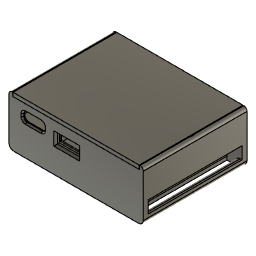
case 8.0 v12 (Autodesk Fusion 360 design; units mm, degrees)
Autodesk Fusion 360 part; units mm, degrees
note: some values were not read from the file. Chosen so that the rebuilt part matches the saved one: which bodies a step acts on; which face or edge a step refers to. Set by a fixed rule: which sketch regions a step uses.
sketch "battery base" plane through (0, 0, 0) normal (0, 0, 1) x (1, 0, 0) in component "case"
  line L0 (0, 0) -> (41, 0)
  line L1 (41, 0) -> (41, 41)
  line L2 (41, 41) -> (0, 41)
  line L3 (0, 41) -> (0, 0)
  dimension "d1" = 41
  dimension "d2" = 41
  constraint horizontal L0
  constraint vertical L1
  constraint horizontal L2
  constraint vertical L3
  constraint coincident L0.start L3.end
  measures "d1" distance of L0.start L2.end
  measures "d2" distance of L0.start L0.end
extrude "Extrude1" add sketch "battery base" along normal blind 8.6 makes body 1 in component "case"
sketch "tray base" plane through (0, 0, 8.6) normal (0, 0, 1) x (-1, 0, 0) in component "case"
  line L0 (0, -41) -> (0, 0)
  line L1 (0, 0) -> (-41, 0)
  line L2 (-41, 0) -> (-41, -41)
  line L3 (-41, -41) -> (0, -41)
  line L4 (-41, -41) -> (-47.5, -41)
  line L5 (-47.5, -41) -> (-47.5, 0)
  line L6 (-47.5, 0) -> (-41, 0)
  line L7 (-20.5, 0) -> (-20.5, -41) construction
  line L8 (6.5, -41) -> (6.5, 0)
  line L9 (6.5, 0) -> (0, 0)
  line L10 (0, -41) -> (6.5, -41)
  point P0 (18.675, 37.8)
  dimension "d5" = 6.5
  constraint coincident L2.end L3.start
  constraint perpendicular L2 L4
  constraint perpendicular L1 L5
  constraint coincident L1.end L2.start
  constraint perpendicular L2 L6
  constraint midpoint L1 L7.start
  constraint midpoint L3 L7.end
  constraint symmetric L2.end L7 L0.start
  constraint symmetric L4.end L7 L8.start
  constraint symmetric L5.end L7 L8.end
  constraint symmetric L1.end L7 L0.end
  measures "d5" distance of L5.end L1.end
extrude "Extrude2" add sketch "tray base" along normal blind 9.8 bodies 1 in component "case"
shell "Shell1" thickness 1.6 outward yes removed faces 1 at (11.5, 13.6667, 18.4) on bodies 1 in component "case"
ref_plane "WorkPlane1" through (20.5, 20.5, 8.4) normal (0, -1, 0) x (1, 0, 0) in component "case"
ref_plane "WorkPlane2" through (20.5, 20.5, 2.7) normal (-1, 0, 0) x (0, -1, 0) in component "case"
sketch "buckle" plane through (0, -1.6, 0) normal (0, -1, 0) x (1, 0, 0) in component "case"
  line L0 (42.6, -1.6) -> (49.1, -1.6) construction
  line L1 (49.1, -1.6) -> (49.1, 7) construction
  line L2 (49.1, 1.8) -> (46.3, 1.8) construction
  line L3 (46.3, 1.8) -> (46.3, -1.6) construction
  line L4 (49.1, 1.8) -> (48.3, 1.8)
  line L5 (46.3, -0.2) -> (46.3, -1.6)
  line L6 (46.3, -1.6) -> (47.1, -1.6)
  line L7 (49.1, 0.4) -> (49.1, 1.8)
  arc A0 (47.1, -1.6) -> (49.1, 0.4) centre (47.1, 0.4) ccw
  arc A1 (48.3, 1.8) -> (46.3, -0.2) centre (48.3, -0.2) ccw
  line L8 (-1.6, -1.6) -> (42.6, -1.6)
  line L9 (42.6, -1.6) -> (42.6, 7)
  line L10 (42.6, 7) -> (49.1, 7)
  line L11 (49.1, 7) -> (49.1, 18.4)
  line L12 (49.1, 18.4) -> (-8.1, 18.4)
  line L13 (-8.1, 18.4) -> (-8.1, 7)
  line L14 (-8.1, 7) -> (-1.6, 7)
  line L15 (-1.6, 7) -> (-1.6, -1.6)
  line L16 (49.1, 1.8) -> (49.1, 7)
  line L17 (42.6, -1.6) -> (42.6, 7)
  line L18 (42.6, 7) -> (49.1, 7)
  arc A2 (49.1, 7) -> (42.6, -0.129) centre (50.5661, -0.8645) ccw
  line L19 (42.6, -1.6) -> (46.3, -1.6)
  dimension "d16" = 2
  dimension "d231" = 8
  dimension "d233" = 3.4
  dimension "d234" = 2.8
  constraint coincident L1.end L10.end
  constraint coincident L1 L2.start
  constraint perpendicular L1 L2
  constraint coincident L0 L3.end
  constraint perpendicular L0 L3
  constraint horizontal L4
  constraint vertical L5
  constraint horizontal L6
  constraint vertical L7
  constraint tangent L6 A0
  constraint tangent L7 A0
  constraint tangent L4 A1
  constraint tangent L5 A1
  constraint equal A0 A1
  constraint coincident L0.start L8.end
  constraint coincident L9.end L10.start
  constraint coincident L9 A2.end
  constraint perpendicular L16 L18
  constraint perpendicular L17 L19
  measures "d16" radius of A0
  measures "d231" radius of A2
  measures "d233" distance of L0 L2
  measures "d234" distance of L1 L3
extrude "Extrude1'" add sketch "buckle" against normal up to surface (22.1 mm away) contours L4 L5 L6 L7 A0 A1 | L4 L5 A1 L9 L16 L17 A2 L19 | L9 L10 L17 L18 A2 bodies 1 in component "case"
extrude "Extrude2'" cut sketch "buckle" along normal blind 20 from surface at -22.1 contours L4 L5 A1 L9 L16 L17 A2 L19 bodies 1 in component "case"
mirror "Mirror1" about plane through (20.5, 20.5, 8.4) normal (0, -1, 0) of "Extrude1'", "Extrude2'" in component "case"
split "Split1" by curves path "buckle" along L17 L18 bodies 1 makes body 2 at (13.1333, 27.1667, -1.6) in component "case"
mirror "Mirror2" about plane through (20.5, 20.5, 2.7) normal (-1, 0, 0) of bodies 1 makes body 3 in component "case"
combine "Combine1" operation add target body 2 tool bodies 1 3 in component "case"
sketch "tray" plane through (0, 0, 0) normal (0, 0, 1) x (1, 0, 0) in component "tray"
  line L0 (0, 41) -> (-6.5, 41) construction
  line L1 (41, 41) -> (0, 41) construction
  line L2 (47.5, 41) -> (41, 41) construction
  line L3 (41, 0) -> (47.5, 0) construction
  line L4 (0, 0) -> (41, 0) construction
  line L5 (-6.5, 0) -> (0, 0) construction
  line L6 (-6.5, 41) -> (-6.5, 0) construction
  line L7 (47.5, 41) -> (47.5, 0) construction
  line L8 (41, 0.15) -> (47.35, 0.15)
  line L9 (47.35, 40.85) -> (47.35, 0.15)
  line L10 (47.35, 40.85) -> (41, 40.85)
  line L11 (41, 40.85) -> (0, 40.85)
  line L12 (0, 40.85) -> (-6.35, 40.85)
  line L13 (-6.35, 40.85) -> (-6.35, 0.15)
  line L14 (-6.35, 0.15) -> (0, 0.15)
  line L15 (0, 0.15) -> (41, 0.15)
  line L16 (10.9, 0.15) -> (10.9, 28.4)
  line L17 (10.9, 28.4) -> (-6.35, 28.4)
  line L18 (11.9, 30.6) -> (11.9, 9.7)
  line L19 (11.9, 9.7) -> (27.9, 9.7)
  line L20 (-6.35, 38.6) -> (17.05, 38.6)
  line L21 (-6.35, 38.6) -> (-6.35, 37.8)
  line L22 (-6.35, 37.8) -> (-2.55, 37.8)
  line L23 (-2.55, 37.8) -> (-2.55, 31.6)
  line L24 (-2.55, 31.6) -> (-1.45, 31.6)
  line L25 (0.45, 30.6) -> (0.45, 27.6)
  line L26 (12.15, 31.6) -> (13.25, 31.6)
  line L27 (13.25, 31.6) -> (13.25, 37.8)
  line L28 (13.25, 37.8) -> (17.05, 37.8)
  line L29 (17.05, 37.8) -> (17.05, 38.6)
  line L30 (0.45, 27.6) -> (10.25, 27.6)
  line L31 (10.25, 27.6) -> (10.25, 30.6)
  line L32 (0.35, 43.6) -> (10.35, 43.6)
  line L33 (0.35, 43.6) -> (0.35, 38.6)
  line L34 (10.35, 43.6) -> (10.35, 38.6)
  line L35 (11.9, 30.6) -> (27.9, 30.6)
  line L36 (27.9, 30.6) -> (27.9, 9.7)
  line L37 (20.95, 0.9) -> (12.05, 0.9)
  line L38 (12.05, 0.9) -> (12.05, 5.9)
  line L39 (12.05, 5.9) -> (20.95, 5.9)
  line L40 (20.95, 5.9) -> (20.95, 0.9)
  line L41 (20.95, 0.9) -> (12.05, 5.9) construction
  line L42 (12.05, 0.9) -> (20.95, 5.9) construction
  line L43 (21.1, 0.75) -> (11.9, 0.75)
  line L44 (11.9, 0.75) -> (11.9, 6.05)
  line L45 (11.9, 6.05) -> (21.1, 6.05)
  line L46 (21.1, 6.05) -> (21.1, 0.75)
  line L47 (2.275, 28.4) -> (2.275, 0.15) construction
  line L48 (7.675, 28.4) -> (-3.125, 28.4)
  line L49 (-3.125, 28.4) -> (-3.125, 26.6)
  line L50 (-3.125, 26.6) -> (7.675, 26.6)
  line L51 (7.675, 26.6) -> (7.675, 28.4)
  line L52 (7.675, 28.4) -> (-3.125, 26.6) construction
  line L53 (-3.125, 28.4) -> (7.675, 26.6) construction
  line L54 (-1.45, 31.6) -> (-1.45, 30.6)
  line L55 (10.25, 30.6) -> (12.15, 30.6)
  line L56 (12.15, 30.6) -> (12.15, 31.6)
  line L57 (-1.45, 30.6) -> (0.45, 30.6)
  line L58 (5.35, 38.6) -> (5.35, 43.6) construction
  line L59 (11.9, 9.7) -> (11.9, 0.15)
  line L60 (12.7, 6.05) -> (12.7, 7.05)
  line L61 (12.7, 7.05) -> (11.9, 7.05)
  line L62 (20.3, 6.05) -> (20.3, 7.05)
  line L63 (22.1, 6.5) -> (22.1, 0.15)
  line L64 (10.9, 28.4) -> (11.9, 28.4)
  line L65 (13.25, 31.6) -> (28.9, 31.6)
  line L66 (28.9, 31.6) -> (28.9, 11.7)
  line L67 (17.05, 38.6) -> (17.05, 40.85)
  line L68 (17.05, 37.8) -> (17.05, 31.6)
  line L69 (21.1, 0.75) -> (21.1, 0.15)
  line L70 (27.9, 28.6) -> (28.9, 28.6)
  line L71 (-1.45, 30.6) -> (-1.45, 28.4)
  line L72 (20.3, 7.05) -> (20.3, 9.7)
  line L73 (0.45, 27.6) -> (-1.45, 27.6)
  line L74 (-1.45, 27.6) -> (-1.45, 28.4)
  line L75 (12.7, 7.05) -> (12.7, 9.7)
  line L76 (11.9, 7.05) -> (10.9, 7.05)
  line L77 (47.35, 40.85) -> (21.7, 40.85)
  line L78 (21.7, 40.85) -> (21.7, 6.5) construction
  line L79 (21.7, 6.5) -> (47.35, 6.5) construction
  line L80 (47.35, 6.5) -> (47.35, 40.85)
  line L81 (21.7, 31.6) -> (21.7, 40.85)
  line L82 (22.1, 6.5) -> (47.35, 6.5)
  line L83 (45.55, 6.5) -> (47.35, 8.3)
  line L84 (45.55, 6.5) -> (48.3393, 6.5) construction
  line L85 (23.5, 6.5) -> (21.7, 8.3)
  line L86 (23.5, 6.5) -> (26.5796, 6.5) construction
  line L87 (21.7, 8.3) -> (21.7, 9.7)
  line L88 (21.7, 31.6) -> (21.7, 30.6)
  line L89 (47.35, 11.7) -> (28.9, 11.7)
  line L90 (28.9, 11.7) -> (27.9, 11.7)
  line L91 (21.7, 35.85) -> (47.35, 35.85)
  line L92 (20.3, 30.6) -> (20.3, 40.85)
  line L93 (22.1, 6.5) -> (21.1, 6.05)
  line L94 (17.05, 38.6) -> (20.3, 38.6)
  line L95 (17.05, 37.8) -> (20.3, 37.8)
  line L96 (18.675, 38.6) -> (18.675, 37.8)
  line L97 (-6.1, 42.6) -> (42.6, 42.6)
  line L98 (13.25, 35.8) -> (17.05, 35.8)
  line L99 (-2.55, 35.8) -> (-6.35, 35.8)
  line L100 (17.05, 35.8) -> (20.3, 35.8)
  point P0 (16.5, 3.4)
  point P1 (2.275, 27.5)
  dimension "d26" = -0.15
  dimension "d32" = 20.9
  dimension "d33" = 16
  dimension "d37" = 23.4
  dimension "d40" = 7
  dimension "d41" = 0.8
  dimension "d44" = 10
  dimension "d63" = 8.9
  dimension "d64" = 5
  dimension "d65" = -0.15
  dimension "d67" = 10.8
  dimension "d68" = 1.8
  dimension "d72" = 1
  dimension "d73" = 11
  dimension "d74" = 9.8
  dimension "d75" = 5
  dimension "d79" = 1
  dimension "d80" = 0.6
  dimension "d81" = 0.8
  dimension "d82" = 1
  dimension "d83" = 0.8
  dimension "d84" = 1
  dimension "d87" = 1
  dimension "d89" = 1
  dimension "d96" = 2
  dimension "d103" = 15.8
  dimension "d104" = 1.1
  dimension "d172" = 45
  dimension "d173" = 1.8
  dimension "d174" = 135
  dimension "d175" = 1.8
  dimension "d177" = 5.2
  dimension "d178" = 5
  dimension "d246" = 17.4
  dimension "d247" = 25.8
  dimension "d248" = 34.5
  dimension "d250" = 1
  dimension "d251" = 2
  dimension "d257" = 28.4
  constraint coincident L15 L16.start
  constraint perpendicular L15 L16
  constraint coincident L13 L17.end
  constraint perpendicular L13 L17
  constraint perpendicular L9 L19
  constraint horizontal L20
  constraint perpendicular L20 L21
  constraint perpendicular L21 L22
  constraint perpendicular L22 L23
  constraint perpendicular L23 L24
  constraint perpendicular L24 L25
  constraint perpendicular L25 L26
  constraint perpendicular L20 L27
  constraint perpendicular L27 L28
  constraint perpendicular L20 L29
  constraint equal L22 L28
  constraint perpendicular L25 L30
  constraint perpendicular L30 L31
  constraint equal L23 L27
  constraint equal L24 L26
  constraint equal L25 L31
  constraint coincident L20 L33.end
  constraint perpendicular L20 L33
  constraint coincident L20 L34.end
  constraint perpendicular L20 L34
  constraint perpendicular L18 L35
  constraint horizontal L37
  constraint perpendicular L37 L38
  constraint parallel L37 L39
  constraint parallel L38 L40
  constraint coincident L41 P0
  constraint coincident L42 P0
  constraint midpoint L17 L47.start
  constraint coincident L15 L47.end
  constraint perpendicular L15 L47
  constraint horizontal L48
  constraint perpendicular L48 L49
  constraint parallel L48 L50
  constraint parallel L49 L51
  constraint coincident L52 P1
  constraint coincident L53 P1
  constraint coincident L47 P1
  constraint collinear L17 L48
  constraint coincident L24 L54.start
  constraint perpendicular L24 L54
  constraint equal L21 L29
  constraint perpendicular L31 L55
  constraint perpendicular L26 L56
  constraint perpendicular L25 L57
  constraint midpoint L20 L58.start
  constraint midpoint L32 L58.end
  constraint perpendicular L32 L58
  constraint equal L55 L57
  constraint coincident L15 L59.end
  constraint perpendicular L15 L59
  constraint collinear L44 L59
  constraint coincident L45 L60.start
  constraint perpendicular L45 L60
  constraint coincident L59 L61.end
  constraint perpendicular L59 L61
  constraint coincident L45 L62.start
  constraint perpendicular L45 L62
  constraint coincident L15 L63.end
  constraint perpendicular L15 L63
  constraint equal L60 L62
  constraint collinear L13 L21
  constraint coincident L18 L64.end
  constraint perpendicular L18 L64
  constraint coincident L11 L67.end
  constraint perpendicular L11 L67
  constraint coincident L65 L68.end
  constraint perpendicular L65 L68
  constraint perpendicular L43 L69
  constraint coincident L36 L70.start
  constraint coincident L66 L70.end
  constraint perpendicular L66 L70
  constraint vertical L71
  constraint coincident L17 L71.end
  constraint coincident L48 L71.end
  constraint coincident L19 L72.end
  constraint perpendicular L19 L72
  constraint perpendicular L71 L73
  constraint perpendicular L48 L74
  constraint coincident L19 L75.end
  constraint perpendicular L19 L75
  constraint coincident L16 L76.end
  constraint perpendicular L16 L76
  constraint horizontal L77
  constraint vertical L78
  constraint horizontal L79
  constraint vertical L80
  constraint perpendicular L65 L66
  constraint coincident L78 L81.start
  constraint coincident L65 L81.start
  constraint coincident L79 L63.start
  constraint coincident L63 L82.start
  constraint horizontal L84
  constraint coincident L79 L83.start
  constraint coincident L9 L83.end
  constraint horizontal L86
  constraint coincident L82 L85.start
  constraint coincident L78 L85.end
  constraint coincident L78 L87.end
  constraint coincident L19 L87.end
  constraint coincident L78 L88.end
  constraint coincident L35 L88.end
  constraint coincident L80 L89.start
  constraint coincident L66 L89.end
  constraint perpendicular L66 L89
  constraint coincident L36 L90.end
  constraint perpendicular L36 L90
  constraint coincident L78 L91.start
  constraint coincident L9 L91.end
  constraint perpendicular L9 L91
  constraint coincident L35 L92.start
  constraint coincident L11 L92.end
  constraint perpendicular L11 L92
  constraint collinear L72 L92
  constraint coincident L92 L94.end
  constraint perpendicular L92 L94
  constraint coincident L92 L95.end
  constraint perpendicular L92 L95
  constraint midpoint L94 L96.start
  constraint midpoint L95 L96.end
  constraint coincident L27 L98.start
  constraint coincident L68 L98.end
  constraint perpendicular L68 L98
  constraint coincident L23 L99.start
  constraint coincident L13 L99.end
  constraint perpendicular L13 L99
  constraint collinear L98 L99
  constraint coincident L92 L100.end
  constraint perpendicular L92 L100
  measures "d32" distance of L18.start L18.end
  measures "d33" distance of L18.end L19.end
  measures "d37" distance of L20.start L20.end
  measures "d40" distance of L20 L24
  measures "d41" distance of L20.start L21.end
  measures "d44" distance of L32.start L32.end
  measures "d63" distance of L38.end L39.end
  measures "d64" distance of L37.end L38.end
  measures "d67" distance of L49.end L50.end
  measures "d68" distance of L48.end L49.end
  measures "d72" distance of L24.end L54.end
  measures "d73" distance of L20 L30
  measures "d74" distance of L25 L31
  measures "d75" distance of L20 L32
  measures "d79" distance of L16 L18
  measures "d80" distance of L15 L43
  measures "d81" distance of L60.end L61.end
  measures "d82" distance of L60.start L60.end
  measures "d83" distance of L46 L62
  measures "d84" distance of L46 L63
  measures "d87" distance of L26 L35
  measures "d89" distance of L36 L66
  measures "d96" distance of L35 L70
  measures "d103" distance of L23 L27
  measures "d104" distance of L23.end L24.end
  measures "d172" angle of L83 L84
  measures "d173" distance of L80 L83.start
  measures "d174" angle of L85 L86
  measures "d175" distance of L78 L85.start
  measures "d177" distance of L82 L89
  measures "d178" distance of L11 L91
  measures "d246" distance of L6 L16
  measures "d247" distance of L7 L78
  measures "d248" distance of L2 L82
  measures "d250" distance of L32 L97
  measures "d251" distance of L22 L99
  measures "d257" distance of L5 L17
extrude "Extrude1''" add sketch "tray" against normal blind 1 separate body contours L15 L46 L63 L69 L93 | L9 L80 L82 L83 | L15 L43 L59 L69 | L19 L45 L62 L72 L82 L85 L87 L93 | L9 L19 L36 L80 L82 L83 L85 L87 L89 L90 | L15 L16 L44 L59 L76 | L43 L44 L45 L46 L59 | L9 L65 L66 L80 L81 L89 L91 | L13 L14 L15 L16 L17 L30 L31 L49 L50 L51 | L19 L45 L60 L62 L72 L75 | L9 L10 L11 L77 L80 L81 L91 | L36 L66 L70 L90 | L16 L18 L59 L64 L76 | L45 L59 L60 L61 | L18 L19 L35 L36 L55 | L11 L65 L81 L92 | L35 L36 L65 L66 L70 L88 | L17 L18 L31 L55 L64 | L19 L59 L61 L75 | L35 L65 L88 L92 | L13 L17 L23 L24 L48 L54 L71 L99 | L17 L30 L31 L51 | L13 L17 L20 L21 L22 L23 L24 L25 L26 L27 L28 L29 L31 L35 L48 L54 L55 L56 L57 | L26 L35 L56 L65 L92 | L65 L68 L92 L100 | L11 L67 L92 L94 | L13 L22 L23 L99 | L17 L30 L48 L49 L50 L51 L73 L74 | L17 L25 L30 L48 L51 | L27 L65 L68 L98 | L68 L92 L95 L100 | L11 L20 L34 L67 | L92 L94 L95 L96 | L17 L25 L48 L57 L71 | L17 L25 L48 L73 L74 | L27 L28 L68 L98 | L11 L20 L33 L34 | L29 L94 L95 L96 | L11 L12 L13 L20 L33 | L37 L38 L39 L40 makes body 4 in component "tray"
extrude "Extrude3" add sketch "tray" along normal blind 3 contours L16 L18 L59 L64 L76 | L11 L65 L81 L92 | L19 L59 L61 L75 | L35 L65 L88 L92 | L13 L17 L23 L24 L48 L54 L71 L99 | L26 L35 L56 L65 L92 | L65 L68 L92 L100 | L11 L67 L92 L94 | L13 L22 L23 L99 | L17 L30 L48 L49 L50 L51 L73 L74 | L27 L65 L68 L98 | L68 L92 L95 L100 | L11 L20 L34 L67 | L92 L94 L95 L96 | L27 L28 L68 L98 | L11 L12 L13 L20 L33 bodies 4 in component "tray"
extrude "Extrude4" add sketch "tray" along normal blind 4.8 contours L15 L46 L63 L69 L93 | L9 L80 L82 L83 | L15 L43 L59 L69 | L19 L45 L62 L72 L82 L85 L87 L93 | L15 L16 L44 L59 L76 | L45 L59 L60 L61 | L11 L65 L81 L92 | L35 L65 L88 L92 bodies 4 in component "tray"
extrude "Extrude7" add sketch "tray" along normal blind 2 contours L35 L36 L65 L66 L70 L88 bodies 4 in component "tray"
extrude "Extrude12" add sketch "tray" along normal blind 3.4 contours L9 L19 L36 L80 L82 L83 L85 L87 L89 L90 bodies 4 in component "tray"
extrude "Extrude11" add sketch "tray" along normal blind 0.8 contours L9 L10 L11 L77 L80 L81 L91 bodies 4 in component "tray"
sketch "jst hole" plane through (0, 0.15, 0) normal (0, -1, 0) x (1, 0, 0) in component "tray"
  line L0 (-6.35, 0) -> (-6.35, -1)
  line L1 (-6.35, -1) -> (22.1, -1)
  line L2 (22.1, -1) -> (22.1, 4.8)
  line L3 (22.1, 4.8) -> (10.9, 4.8)
  line L4 (10.9, 4.8) -> (10.9, 0)
  line L5 (16.5, 0) -> (16.5, 4.8) construction
  line L6 (21.05, 0) -> (11.95, 0)
  line L7 (11.95, 0) -> (11.95, 4.1)
  line L8 (11.95, 4.1) -> (21.05, 4.1)
  line L9 (21.05, 4.1) -> (21.05, 0)
  line L10 (21.05, 0) -> (11.95, 4.1) construction
  line L11 (11.95, 0) -> (21.05, 4.1) construction
  line L12 (11.95, 0.6) -> (21.05, 0.6)
  line L13 (11.95, 3.5) -> (21.05, 3.5)
  line L14 (15.5, 4.8) -> (15.5, 4.1)
  line L15 (17.5, 4.8) -> (17.5, 4.1)
  line L16 (15.5, 4.1) -> (17.5, 4.8) construction
  line L17 (-6.35, 0) -> (10.9, 0)
  point P0 (16.5, 2.05)
  point P1 (16.5, 4.45)
  dimension "d132" = 9.1
  dimension "d133" = 4.1
  dimension "d134" = 0.6
  dimension "d135" = 0.6
  dimension "d138" = 2
  constraint midpoint L3 L5.end
  constraint horizontal L6
  constraint perpendicular L6 L7
  constraint parallel L6 L8
  constraint parallel L7 L9
  constraint coincident L10 P0
  constraint coincident L11 P0
  constraint coincident L5 P0
  constraint coincident L7 L12.start
  constraint coincident L9 L12.end
  constraint perpendicular L9 L12
  constraint coincident L7 L13.start
  constraint coincident L9 L13.end
  constraint perpendicular L9 L13
  constraint coincident L3 L14.start
  constraint coincident L8 L14.end
  constraint perpendicular L8 L14
  constraint coincident L3 L15.start
  constraint coincident L8 L15.end
  constraint perpendicular L8 L15
  constraint midpoint L16 P1
  constraint coincident L5 P1
  constraint collinear L6 L17
  constraint perpendicular L5 L6
  measures "d132" distance of L7.end L8.end
  measures "d133" distance of L6.end L7.end
  measures "d134" distance of L6 L12
  measures "d135" distance of L8 L13
  measures "d138" distance of L14 L15
extrude "Extrude9" cut sketch "jst hole" along normal through all from surface at -0.6 contours L7 L9 L12 L13 bodies 4 in component "tray"
extrude "Extrude10" add sketch "jst hole" against normal blind 0.8 from surface at -0.6 contours L3 L8 L14 L15 bodies 4 in component "tray"
chamfer "Chamfer1" distance 0.7 distance2 0.8 1 edges at (16.5, 1.55, 4.8) measured on face at (16.1667, 1.55, 4.5667) on bodies 4 in component "tray"
extrude "Extrude13" add sketch "tray" along normal blind 1.5 from surface at 4.8 contours L9 L80 L82 L83 | L19 L45 L62 L72 L82 L85 L87 L93 | L11 L65 L81 L92 | L35 L65 L88 L92 bodies 4 in component "tray"
sketch "usb-c and jst holes" plane through (0, 0, 0) normal (0, 1, 0) x (-1, 0, 0) in component "case"
  line L0 (-41, 0) -> (0, 0)
  line L1 (0, 0) -> (0, 8.6)
  line L2 (0, 8.6) -> (6.5, 8.6)
  line L3 (6.5, 8.6) -> (6.5, 18.4)
  line L4 (-47.5, 18.4) -> (-47.5, 8.6)
  line L5 (-47.5, 8.6) -> (-41, 8.6)
  line L6 (-41, 8.6) -> (-41, 0)
  line L7 (6.35, 9.6) -> (-10.9, 9.6)
  line L8 (-10.9, 9.6) -> (-10.9, 14.4)
  line L9 (6.5, 8.6) -> (6.5, 18.4)
  line L10 (6.5, 9.9297) -> (-10.9, 9.9297) construction
  line L11 (1.0582, 11.4) -> (-5.5418, 11.4)
  line L12 (-6.8418, 12.7) -> (-6.8418, 13.9)
  line L13 (-5.5418, 15.2) -> (1.0582, 15.2)
  line L14 (2.3582, 13.9) -> (2.3582, 12.7)
  line L15 (2.3582, 11.4) -> (-6.8418, 15.2) construction
  line L16 (-6.8418, 11.4) -> (2.3582, 15.2) construction
  line L17 (-2.2, 9.9297) -> (-2.2951, 17.6) construction
  arc A0 (-5.5418, 15.2) -> (-6.8418, 13.9) centre (-5.5418, 13.9) ccw
  arc A1 (2.3582, 13.9) -> (1.0582, 15.2) centre (1.0582, 13.9) ccw
  arc A2 (1.0582, 11.4) -> (2.3582, 12.7) centre (1.0582, 12.7) ccw
  arc A3 (-6.8418, 12.7) -> (-5.5418, 11.4) centre (-5.5418, 12.7) ccw
  line L18 (6.5, 18.4) -> (-47.5, 18.4)
  line L19 (-11.95, 10.2) -> (-11.95, 13.1)
  line L20 (-21.05, 10.2) -> (-11.95, 10.2)
  line L21 (-11.95, 13.1) -> (-21.05, 13.1)
  line L22 (-21.05, 13.1) -> (-21.05, 10.2)
  line L23 (-11.8, 13.7) -> (-11.8, 10.2)
  line L24 (-11.8, 10.2) -> (-11.95, 10.2)
  line L25 (-16.5, 13.1) -> (-16.5, 13.7)
  line L26 (-16.5, 13.7) -> (-11.8, 13.7)
  line L27 (-16.5, 13.7) -> (-21.2, 13.7)
  line L28 (-21.2, 13.7) -> (-21.2, 10.2)
  line L29 (-21.2, 10.2) -> (-21.05, 10.2)
  line L30 (-21.2, 10.2) -> (-21.2, 9.6)
  line L31 (-21.2, 9.6) -> (-11.8, 9.6)
  line L32 (-11.8, 9.6) -> (-11.8, 10.2)
  point P0 (-2.2418, 13.3)
  dimension "d145" = 9.2
  dimension "d146" = 3.8
  dimension "d149" = 1.8
  dimension "d150" = 1.3
  dimension "d187" = 0.6
  dimension "d188" = 0.15
  dimension "d249" = 0.6
  constraint coincident L9 L10.start
  constraint coincident L8 L10.end
  constraint perpendicular L8 L10
  constraint horizontal L11
  constraint perpendicular L11 L12
  constraint parallel L11 L13
  constraint parallel L12 L14
  constraint coincident L15 P0
  constraint coincident L16 P0
  constraint midpoint L10 L17.start
  constraint coincident P0 L17
  constraint coincident L15.end L12
  constraint coincident L15.end L13
  constraint tangent L12 A0
  constraint tangent L13 A0
  constraint coincident L16.end L13
  constraint coincident L16.end L14
  constraint tangent L13 A1
  constraint tangent L14 A1
  constraint equal A0 A1
  constraint coincident L15.start L14
  constraint coincident L15.start L11
  constraint tangent L14 A2
  constraint tangent L11 A2
  constraint equal A0 A2
  constraint coincident L16.start L11
  constraint coincident L16.start L12
  constraint tangent L11 A3
  constraint tangent L12 A3
  constraint equal A0 A3
  constraint perpendicular L20 L23
  constraint coincident L19.start L20.end
  constraint perpendicular L19 L24
  constraint midpoint L21 L25.start
  constraint perpendicular L21 L25
  constraint coincident L23 L26.end
  constraint perpendicular L23 L26
  constraint symmetric L23.end L25 L28.end
  constraint symmetric L19.start L25 L20.start
  constraint symmetric L26.start L25 L27.start
  constraint symmetric L25 L23.start L27.end
  constraint perpendicular L29 L30
  constraint perpendicular L23 L31
  constraint perpendicular L24 L32
  measures "d145" distance of L15.end L16.end
  measures "d146" distance of L15.start L16.end
  measures "d149" distance of L7 L11
  measures "d150" radius of A0
  measures "d187" distance of L25.start L25.end
  measures "d188" distance of L23.end L19.start
  measures "d249" distance of L28.end L30.end
extrude "Extrude3'" cut sketch "usb-c and jst holes" against normal through all contours L11 L12 L13 L14 A0 A1 A2 A3 | L19 L20 L21 L22 | L20 L24 L29 L30 L31 L32 | L19 L21 L23 L24 L25 L26 | L21 L22 L25 L27 L28 L29 bodies 2 in component "case"
chamfer "Chamfer3" distance 0.6 angle 45 16 edges at (6.461, 0, 11.7808) (6.8418, 0, 13.3) (6.461, 0, 14.8192) (2.2418, 0, 15.2) (-1.9774, 0, 14.8192) (-2.3582, 0, 13.3) (-1.9774, 0, 11.7808) (2.2418, 0, 11.4) (6.461, -1.6, 11.7808) (2.2418, -1.6, 11.4) (-1.9774, -1.6, 11.7808) (-2.3582, -1.6, 13.3) (-1.9774, -1.6, 14.8192) (2.2418, -1.6, 15.2) (6.461, -1.6, 14.8192) (6.8418, -1.6, 13.3) on bodies 2 in component "case"
chamfer "Chamfer4" distance 0.8 angle 45 4 edges at (21.2, -1.6, 11.65) (16.5, -1.6, 13.7) (11.8, -1.6, 11.65) (16.5, -1.6, 9.6) on bodies 2 in component "case"
sketch "switch hole" plane through (0, 41, 0) normal (0, -1, 0) x (1, 0, 0) in component "case"
  line L0 (0, 0) -> (41, 0)
  line L1 (41, 0) -> (41, 8.6)
  line L2 (41, 8.6) -> (47.5, 8.6)
  line L3 (47.5, 8.6) -> (47.5, 18.4)
  line L4 (-6.5, 18.4) -> (-6.5, 8.6)
  line L5 (-6.5, 8.6) -> (0, 8.6)
  line L6 (0, 8.6) -> (0, 0)
  line L7 (10.35, 9.6) -> (0.35, 9.6)
  line L8 (10.35, 9.6) -> (10.35, 12.6)
  line L9 (0.35, 9.6) -> (0.35, 12.6)
  line L10 (5.35, 9.6) -> (5.1215, 17.5967) construction
  line L11 (9.9486, 15.5) -> (0.5486, 15.5)
  line L12 (0.5486, 15.5) -> (0.5486, 10.8)
  line L13 (0.5486, 10.8) -> (9.9486, 10.8)
  line L14 (9.9486, 10.8) -> (9.9486, 15.5)
  line L15 (9.9486, 15.5) -> (0.5486, 10.8) construction
  line L16 (0.5486, 15.5) -> (9.9486, 10.8) construction
  line L17 (47.5, 18.4) -> (-6.5, 18.4)
  point P0 (5.2486, 13.15)
  dimension "d154" = 9.4
  dimension "d155" = 4.7
  dimension "d156" = 1.2
  constraint midpoint L7 L10.start
  constraint horizontal L11
  constraint perpendicular L11 L12
  constraint parallel L11 L13
  constraint parallel L12 L14
  constraint coincident L15 P0
  constraint coincident L16 P0
  constraint coincident L10 P0
  measures "d154" distance of L12.end L13.end
  measures "d155" distance of L11.end L12.end
  measures "d156" distance of L7 L13
extrude "Extrude5" cut sketch "switch hole" against normal through all contours L11 L12 L13 L14 bodies 2 in component "case"
chamfer "Chamfer2" distance 1 angle 45 4 edges at (5.2486, 42.6, 10.8) (9.9486, 42.6, 13.15) (5.2486, 42.6, 15.5) (0.5486, 42.6, 13.15) on bodies 2 in component "case"
sketch "switch keyhole" plane through (0, 0, 18.4) normal (0, 0, 1) x (-1, 0, 0) in component "case"
  line L0 (6.5, 0) -> (6.5, -41)
  line L1 (6.5, -41) -> (-47.5, -41)
  line L2 (-47.5, -41) -> (-47.5, 0)
  line L3 (-47.5, 0) -> (6.5, 0)
  line L4 (-49.1, -42.6) -> (8.1, -42.6)
  line L5 (8.1, -42.6) -> (8.1, 1.6)
  line L6 (8.1, 1.6) -> (-49.1, 1.6)
  line L7 (-49.1, 1.6) -> (-49.1, -42.6)
  line L8 (-9.9486, -41) -> (-9.9486, -41.6)
  line L9 (-0.5486, -41) -> (-0.5486, -41.6)
  line L10 (-9.9486, -41.6) -> (-0.5486, -41.6) construction
  line L11 (-5.2486, -41.6) -> (-5.2486, -42.6) construction
  line L12 (-8.2486, -41) -> (-8.2486, -42.6)
  line L13 (-2.2486, -41) -> (-2.2486, -42.6)
  line L14 (-2.2486, -42.6) -> (-8.2486, -41) construction
  point P0 (-5.2486, -41.8)
  dimension "d159" = 6
  constraint coincident L8.end L10.start
  constraint coincident L9.end L10.end
  constraint midpoint L10 L11.start
  constraint coincident L4 L11.end
  constraint perpendicular L4 L11
  constraint coincident L1 L12.start
  constraint coincident L4 L12.end
  constraint perpendicular L4 L12
  constraint coincident L1 L13.start
  constraint coincident L4 L13.end
  constraint perpendicular L4 L13
  constraint midpoint L14 P0
  constraint coincident L11 P0
  measures "d159" distance of L12 L13
extrude "Extrude6" cut sketch "switch keyhole" against normal up to surface (2.9 mm away) contours L1 L4 L12 L13 bodies 2 in component "case"
sketch "usb-b" plane through (0, 41, 0) normal (0, -1, 0) x (1, 0, 0) in component "case"
  line L0 (2.2486, 18.4) -> (-6.5, 18.4)
  line L1 (-6.5, 18.4) -> (-6.5, 8.6)
  line L2 (-6.5, 8.6) -> (0, 8.6)
  line L3 (0, 8.6) -> (0, 0)
  line L4 (0, 0) -> (41, 0)
  line L5 (41, 0) -> (41, 8.6)
  line L6 (41, 8.6) -> (47.5, 8.6)
  line L7 (47.5, 8.6) -> (47.5, 18.4)
  line L8 (47.35, 10.4) -> (21.7, 10.4)
  line L9 (21.7, 10.4) -> (21.7, 15.9)
  line L10 (21.7, 15.9) -> (47.5, 15.9) construction
  line L11 (39.1, 10.4) -> (39.1, 13.6)
  line L12 (39.1, 13.6) -> (31.1, 13.6)
  line L13 (31.1, 13.6) -> (31.1, 10.4)
  line L14 (31.1, 13.6) -> (39.1, 10.4) construction
  line L15 (40.3, 15.2) -> (29.9, 15.2)
  line L16 (29.9, 15.2) -> (29.9, 8.8)
  line L17 (29.9, 8.8) -> (40.3, 8.8)
  line L18 (40.3, 8.8) -> (40.3, 15.2)
  line L19 (40.3, 15.2) -> (29.9, 8.8) construction
  line L20 (29.9, 15.2) -> (40.3, 8.8) construction
  line L21 (2.2486, 15.5) -> (2.2486, 18.4)
  line L22 (47.5, 18.4) -> (8.2486, 18.4)
  line L23 (8.2486, 18.4) -> (8.2486, 15.5)
  line L24 (8.2486, 15.5) -> (9.9486, 15.5)
  line L25 (9.9486, 15.5) -> (9.9486, 10.8)
  line L26 (9.9486, 10.8) -> (0.5486, 10.8)
  line L27 (0.5486, 10.8) -> (0.5486, 15.5)
  line L28 (0.5486, 15.5) -> (2.2486, 15.5)
  point P0 (35.1, 12)
  dimension "d191" = 9.4
  dimension "d192" = 8.4
  dimension "d193" = 3.2
  dimension "d195" = 10.4
  dimension "d196" = 6.4
  constraint coincident L9.end L10.start
  constraint coincident L7 L10.end
  constraint perpendicular L7 L10
  constraint coincident L8 L11.start
  constraint perpendicular L8 L11
  constraint perpendicular L11 L12
  constraint coincident L8 L13.end
  constraint perpendicular L8 L13
  constraint horizontal L15
  constraint perpendicular L15 L16
  constraint parallel L15 L17
  constraint parallel L16 L18
  constraint coincident L19 P0
  constraint coincident L20 P0
  constraint midpoint L14 P0
  measures "d191" distance of L9 L13
  measures "d192" distance of L7 L11
  measures "d193" distance of L8 L12
  measures "d195" distance of L16.end L17.end
  measures "d196" distance of L15.end L16.end
extrude "Extrude8" cut sketch "usb-b" against normal through all contours L8 L11 L12 L13 bodies 2 in component "case"
extrude "Extrude9'" cut sketch "usb-b" against normal through all from surface at -0.6 contours L8 L16 L17 L18 | L8 L11 L12 L13 L15 L16 L18 bodies 2 in component "case"
sketch "lid 0" plane through (0, 0, 0) normal (0, 0, 1) x (1, 0, 0) in component "lid"
  line L0 (-8.1, 42.6) -> (-8.1, -1.6) construction
  line L1 (2.2486, 42.6) -> (-8.1, 42.6)
  line L2 (49.1, -1.6) -> (49.1, 42.6) construction
  line L3 (49.1, 42.6) -> (8.2486, 42.6)
  line L4 (-8.1, -1.6) -> (49.1, -1.6)
  line L5 (-6.5, 41) -> (2.2486, 41)
  line L6 (-6.5, 0) -> (-6.5, 41) construction
  line L7 (47.5, 0) -> (-6.5, 0)
  line L8 (47.5, 41) -> (47.5, 0) construction
  line L9 (8.2486, 41) -> (47.5, 41)
  line L10 (2.2486, 41) -> (2.2486, 42.6)
  line L11 (8.2486, 42.6) -> (8.2486, 41)
  line L12 (8.2486, 42.6) -> (2.2486, 42.6)
  line L13 (-6.35, 42.6) -> (-6.35, -1.6)
  line L14 (47.35, 42.6) -> (47.35, -1.6)
  line L15 (-6.35, 40.85) -> (2.3986, 40.85)
  line L16 (2.3986, 40.85) -> (2.3986, 42.6)
  line L17 (8.0986, 42.6) -> (8.0986, 40.85)
  line L18 (8.0986, 40.85) -> (47.35, 40.85)
  line L19 (-6.35, 0.15) -> (47.35, 0.15)
  line L20 (-6.35, 0.95) -> (47.35, 0.95)
  line L21 (-6.35, 40.05) -> (47.35, 40.05)
  line L22 (47.35, 38.85) -> (46.55, 38.85)
  line L23 (46.55, 38.85) -> (46.55, 40.05)
  line L24 (47.35, 20.5) -> (-6.35, 20.5) construction
  line L25 (46.55, 2.15) -> (46.55, 0.95)
  line L26 (47.35, 2.15) -> (46.55, 2.15)
  line L27 (20.5, 0.95) -> (20.5, 40.05) construction
  line L28 (-6.35, 2.15) -> (-5.55, 2.15)
  line L29 (-5.55, 2.15) -> (-5.55, 0.95)
  line L30 (-6.35, 38.85) -> (-5.55, 38.85)
  line L31 (-5.55, 38.85) -> (-5.55, 40.05)
  dimension "d202" = 0.15
  dimension "d203" = 0.15
  dimension "d204" = 0.8
  dimension "d205" = 0.8
  dimension "d206" = 0.15
  dimension "d207" = 0.15
  dimension "d208" = 0.15
  dimension "d209" = 0.15
  dimension "d212" = 0.8
  dimension "d213" = 1.2
  constraint coincident L3.end L11.start
  constraint coincident L1.start L10.end
  constraint coincident L1 L13.start
  constraint coincident L4 L13.end
  constraint perpendicular L4 L13
  constraint coincident L3 L14.start
  constraint coincident L4 L14.end
  constraint perpendicular L4 L14
  constraint coincident L13 L15.start
  constraint perpendicular L13 L15
  constraint coincident L12 L16.end
  constraint perpendicular L12 L16
  constraint coincident L12 L17.start
  constraint perpendicular L12 L17
  constraint coincident L14 L18.end
  constraint perpendicular L14 L18
  constraint coincident L13 L19.start
  constraint coincident L14 L19.end
  constraint perpendicular L14 L19
  constraint coincident L13 L20.start
  constraint coincident L14 L20.end
  constraint perpendicular L14 L20
  constraint coincident L13 L21.start
  constraint coincident L14 L21.end
  constraint perpendicular L8 L21
  constraint collinear L15 L18
  constraint coincident L14 L22.start
  constraint perpendicular L14 L22
  constraint coincident L21 L23.end
  constraint perpendicular L21 L23
  constraint midpoint L14 L24.start
  constraint midpoint L13 L24.end
  constraint symmetric L22.start L24 L26.start
  constraint symmetric L22.end L24 L25.start
  constraint symmetric L23.end L24 L25.end
  constraint midpoint L20 L27.start
  constraint midpoint L21 L27.end
  constraint symmetric L22.start L27 L30.start
  constraint symmetric L22.end L27 L30.end
  constraint symmetric L23.end L27 L31.end
  constraint symmetric L25.start L27 L28.end
  constraint symmetric L25.end L27 L29.end
  constraint symmetric L26.start L27 L28.start
  measures "d202" distance of L6 L13
  measures "d203" distance of L8 L14
  measures "d204" distance of L15 L21
  measures "d205" distance of L19 L20
  measures "d206" distance of L5 L15
  measures "d207" distance of L10 L16
  measures "d208" distance of L11 L17
  measures "d209" distance of L7 L19
  measures "d212" distance of L22.start L22.end
  measures "d213" distance of L22.end L23.end
extrude "Extrude1'''" add sketch "lid 0" along normal blind 1.6 separate body makes body 5 in component "lid"
extrude "Extrude2''" add sketch "lid 0" against normal blind 1.6 contours L12 L13 L14 L15 L16 L17 L18 L21 | L13 L21 L30 L31 | L14 L21 L22 L23 | L13 L20 L28 L29 | L13 L14 L19 L20 | L14 L20 L25 L26 bodies 5 in component "lid"
sketch "Sketch4" plane through (0, 0, 18.4) normal (0, 0, 1) x (-1, 0, 0) in component "case"
  line L0 (-2.2486, -42.6) -> (8.1, -42.6)
  line L1 (8.1, -42.6) -> (8.1, 1.6)
  line L2 (8.1, 1.6) -> (-49.1, 1.6)
  line L3 (-49.1, 1.6) -> (-49.1, -42.6)
  line L4 (-47.5, -41) -> (-47.5, 0)
  line L5 (-47.5, 0) -> (6.5, 0)
  line L6 (6.5, 0) -> (6.5, -41)
  line L7 (-8.2486, -41) -> (-47.5, -41)
  line L8 (-8.2486, -41) -> (-8.2486, -42.6)
  line L9 (6.5, 0) -> (6.5, 1.6)
  line L10 (-47.5, 0) -> (-47.5, 1.6)
  line L11 (-47.5, -41) -> (-47.5, -42.6)
  line L12 (-2.2486, -41) -> (-2.2486, -42.6)
  line L13 (-49.1, -42.6) -> (-8.2486, -42.6)
  line L14 (-8.2486, -42.6) -> (-8.2486, -41)
  line L15 (6.5, -41) -> (6.5, -42.6)
  line L16 (6.5, -41) -> (-2.2486, -41)
  constraint coincident L7.start L8.start
  constraint coincident L0 L8.end
  constraint perpendicular L0 L8
  constraint coincident L5.end L6.start
  constraint coincident L2 L9.end
  constraint perpendicular L2 L9
  constraint coincident L4.end L5.start
  constraint coincident L2 L10.end
  constraint perpendicular L2 L10
  constraint coincident L4.start L7.end
  constraint coincident L6.end L15.start
  constraint coincident L0 L15.end
  constraint perpendicular L0 L15
extrude "Extrude10'" add sketch "Sketch4" along normal blind 1.6 contours L0 L1 L2 L6 L9 L15 | L2 L3 L4 L10 L11 L13 bodies 2 in component "case"
sketch "nubs" plane through (47.35, 0, 0) normal (1, 0, 0) x (0, 1, 0)
  line L0 (40.85, 18.4) -> (42.6, 18.4)
  line L1 (42.6, 20) -> (-1.6, 20)
  line L2 (-1.6, 20) -> (-1.6, 18.4)
  line L3 (0.15, 18.4) -> (0.15, 16.8)
  line L4 (0.15, 16.8) -> (2.15, 16.8)
  line L5 (2.15, 16.8) -> (2.15, 18.4)
  line L6 (38.85, 18.4) -> (38.85, 16.8)
  line L7 (38.85, 16.8) -> (40.85, 16.8)
  line L8 (40.85, 16.8) -> (40.85, 18.4)
  line L9 (20.5, 20) -> (20.5, 18.4) construction
  line L10 (21.3, 18.9) -> (19.7, 18.9)
  line L11 (19.7, 18.9) -> (19.7, 19.5)
  line L12 (19.7, 19.5) -> (21.3, 19.5)
  line L13 (21.3, 19.5) -> (21.3, 18.9)
  line L14 (21.3, 18.9) -> (19.7, 19.5) construction
  line L15 (19.7, 18.9) -> (21.3, 19.5) construction
  line L16 (42.6, 18.4) -> (42.6, 20)
  line L17 (-1.6, 18.4) -> (0.15, 18.4)
  line L18 (2.15, 18.4) -> (38.85, 18.4)
  point P0 (20.5, 19.2)
  dimension "d220" = 1.6
  dimension "d221" = 0.6
  constraint midpoint L1 L9.start
  constraint horizontal L10
  constraint perpendicular L10 L11
  constraint parallel L10 L12
  constraint parallel L11 L13
  constraint coincident L14 P0
  constraint coincident L15 P0
  constraint midpoint L9 P0
  measures "d220" distance of L11.end L12.end
  measures "d221" distance of L10.end L11.end
extrude "Extrude3''" add sketch "nubs" along normal blind 0.35 contours L10 L11 L12 L13 sketch seen with x (1, 0, 0) y (0, 1, 0) z (0, 0, 1) at (0, 0, -18.4) bodies 5 in component "lid"
mirror "Mirror1'" about plane through (20.5, 20.5, -15.7) normal (-1, 0, 0) of "Extrude3''" in component "lid"
combine "Combine2" operation cut target body 2 tool bodies 5 body 5 seen with x (1, 0, 0) y (0, 1, 0) z (0, 0, 1) at (0, 0, 18.4) keep tools in component "case"
move_face "OffsetFaces1" offset -0.2 10 faces at (47.5667, 20.7667, 18.9) (47.5667, 19.7, 19.1) (47.5667, 20.2333, 19.5) (47.5667, 21.3, 19.3) (47.7, 20.2333, 19.3) (-6.5667, 20.7667, 18.9) (-6.6333, 19.7, 19.1) (-6.6333, 21.3, 19.3) (-6.5667, 20.2333, 19.5) (-6.7, 20.2333, 19.3) on bodies 2 in component "case"
fillet "Fillet1" radius 0.25 2 faces at (47.7, 20.2333, 0.9) (-6.7, 20.2333, 0.9) on bodies 5 in component "lid"
fillet "Fillet1'" radius 1.4 2 edges at (-8.1, 20.5, 20) (49.1, 20.5, 20) on bodies 2 in component "case"
sketch "Sketch5" plane through (-6.5, 0, 0) normal (1, 0, 0) x (0, 1, 0) in component "case"
  line L0 (21.5, 19.7) -> (21.5, 18.7)
  line L1 (21.5, 18.7) -> (19.5, 18.7)
  line L2 (19.5, 18.7) -> (19.5, 19.7)
  line L3 (19.5, 19.7) -> (21.5, 19.7)
  line L4 (0, 8.6) -> (41, 8.6)
  line L5 (41, 8.6) -> (41, 18.4)
  line L6 (41, 18.4) -> (42.6, 18.4)
  line L7 (42.6, 18.4) -> (42.6, 20)
  line L8 (42.6, 20) -> (-1.6, 20)
  line L9 (-1.6, 20) -> (-1.6, 18.4)
  line L10 (-1.6, 18.4) -> (0, 18.4)
  line L11 (0, 18.4) -> (0, 8.6)
  line L12 (28.4, 9.6) -> (0.15, 9.6)
  line L13 (3.2, 12) -> (3.2, 16.4)
  arc A0 (3.2, 16.4) -> (1.6, 16.4) centre (2.4, 16.4) ccw
  line L14 (1.6, 16.4) -> (1.6, 12)
  arc A1 (1.6, 12) -> (3.2, 12) centre (2.4, 12) ccw
  line L15 (2.4, 11.2) -> (2.4, 17.2) construction
  arc A2 (6.2, 16.4) -> (4.6, 16.4) centre (5.4, 16.4) ccw
  line L16 (6.2, 12) -> (6.2, 16.4)
  arc A3 (4.6, 12) -> (6.2, 12) centre (5.4, 12) ccw
  line L17 (4.6, 16.4) -> (4.6, 12)
  arc A4 (9.2, 16.4) -> (7.6, 16.4) centre (8.4, 16.4) ccw
  line L18 (9.2, 12) -> (9.2, 16.4)
  arc A5 (7.6, 12) -> (9.2, 12) centre (8.4, 12) ccw
  line L19 (7.6, 16.4) -> (7.6, 12)
  arc A6 (12.2, 16.4) -> (10.6, 16.4) centre (11.4, 16.4) ccw
  line L20 (12.2, 12) -> (12.2, 16.4)
  arc A7 (10.6, 12) -> (12.2, 12) centre (11.4, 12) ccw
  line L21 (10.6, 16.4) -> (10.6, 12)
  arc A8 (15.2, 16.4) -> (13.6, 16.4) centre (14.4, 16.4) ccw
  line L22 (15.2, 12) -> (15.2, 16.4)
  arc A9 (13.6, 12) -> (15.2, 12) centre (14.4, 12) ccw
  line L23 (13.6, 16.4) -> (13.6, 12)
  arc A10 (18.2, 16.4) -> (16.6, 16.4) centre (17.4, 16.4) ccw
  line L24 (18.2, 12) -> (18.2, 16.4)
  arc A11 (16.6, 12) -> (18.2, 12) centre (17.4, 12) ccw
  line L25 (16.6, 16.4) -> (16.6, 12)
  arc A12 (21.2, 16.4) -> (19.6, 16.4) centre (20.4, 16.4) ccw
  line L26 (21.2, 12) -> (21.2, 16.4)
  arc A13 (19.6, 12) -> (21.2, 12) centre (20.4, 12) ccw
  line L27 (19.6, 16.4) -> (19.6, 12)
  arc A14 (24.2, 16.4) -> (22.6, 16.4) centre (23.4, 16.4) ccw
  line L28 (24.2, 12) -> (24.2, 16.4)
  arc A15 (22.6, 12) -> (24.2, 12) centre (23.4, 12) ccw
  line L29 (22.6, 16.4) -> (22.6, 12)
  arc A16 (27.2, 16.4) -> (25.6, 16.4) centre (26.4, 16.4) ccw
  line L30 (27.2, 12) -> (27.2, 16.4)
  arc A17 (25.6, 12) -> (27.2, 12) centre (26.4, 12) ccw
  line L31 (25.6, 16.4) -> (25.6, 12)
  point P0 (26.6, 12.6)
  dimension "d235" = 1.6
  dimension "d236" = 6
  dimension "d237" = 1.6
  dimension "d238" = 1.6
  dimension "d241" = -3
  dimension "d242" = 0
  constraint tangent L13 A0
  constraint tangent A0 L14
  constraint parallel L13 L14
  constraint tangent L14 A1
  constraint tangent L13 A1
  constraint midpoint A1 L15.start
  constraint midpoint A0 L15.end
  constraint parallel L11 L15
  measures "d235" diameter of A0
  measures "d236" distance of L15.start L15.end
  measures "d237" distance of L12 L15.start
  measures "d238" distance of L11 L14
extrude "Extrude11'" cut sketch "Sketch5" against normal through all contours L13 A0 L14 A1 | A2 L16 A3 L17 | A4 L18 A5 L19 | A6 L20 A7 L21 | A8 L22 A9 L23 | A10 L24 A11 L25 | A12 L26 A13 L27 | A14 L28 A15 L29 | A16 L30 A17 L31 bodies 2 in component "case"
chamfer "Chamfer1'" distance 1.2 distance2 1.6 4 edges at (46.95, 2.15, -1.6) (46.95, 38.85, -1.6) (-5.95, 38.85, -1.6) (-5.95, 2.15, -1.6) measured on face at (11.8167, 0.4167, -1.6) measured on face at (6.1986, 41.4333, -1.6) measured on face at (6.1986, 41.4333, -1.6) measured on face at (11.8167, 0.4167, -1.6) on bodies 5 in component "lid"
extrude "Extrude14" add sketch "tray" along normal blind 5 contours L11 L67 L92 L94 | L13 L22 L23 L99 | L68 L92 L95 L100 | L11 L20 L34 L67 | L27 L28 L68 L98 | L11 L12 L13 L20 L33 bodies 4 in component "tray"
chamfer "Chamfer2'" distance 2 angle 45 2 edges at (-2.55, 36.8, 5) (13.25, 36.8, 5) on bodies 4 in component "tray"
component "case" placed x (1, 0, 0) y (0, 1, 0) z (0, 0, 1) at (0, 0, 0)
component "tray" placed x (1, 0, 0) y (0, 1, 0) z (0, 0, 1) at (0, 0, 9.6)
component "lid" placed x (1, 0, 0) y (0, 1, 0) z (0, 0, 1) at (0, 0, 18.4)
equation "d83 = d81"
equation "d84 = d79"
equation "d87 = d72"
equation "d89 = d87"
equation "d205 = d204"
equation "d207 = d206"
equation "d208 = d207"
named bodies: "case", "case (1) (1)", "case (1)"
